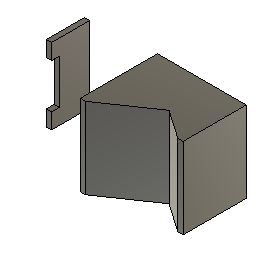
camera_enclosure v9 (Autodesk Fusion 360 design; units mm, degrees)
Autodesk Fusion 360 part; units mm, degrees
sketch "Esboço1" plane through (0, 0, 0) normal (0, 0, 1) x (1, 0, 0)
sketch "Esboço2" plane through (0, 0, 0) normal (0, 0, 1) x (1, 0, 0)
sketch "Esboço3" plane through (0, 0, 0) normal (0, 0, 1) x (1, 0, 0)
  line L0 (13, 0) -> (13, 15)
  line L1 (13, 15) -> (-13, 15)
  line L2 (-13, 15) -> (-13, 0)
  line L3 (-13, 0) -> (-13, -12)
  line L4 (-13, -12) -> (13, -12)
  line L5 (13, -12) -> (13, 0)
  constraint perpendicular L0 L1
  constraint perpendicular L3 L4
sketch "Esboço4" plane through (0, 240.56, 0) normal (0, 1, 0) x (-1, 0, 0)
  arc A0 (-80.638, 38.94) -> (-82.638, 40.94) centre (-82.638, 38.94) ccw
  line L0 (-82.638, 40.94) -> (-88.7191, 40.94)
  arc A1 (-91.2809, 40.94) -> (-88.7191, 40.94) centre (-90, 38.94) ccw
  line L1 (-91.2809, 40.94) -> (-101.2191, 40.94)
  arc A2 (-104.5, 37.6591) -> (-101.2191, 40.94) centre (-102.5, 38.94) ccw
  line L2 (-104.5, 37.6591) -> (-104.5, 19.2209)
  arc A3 (-101.2191, 15.94) -> (-104.5, 19.2209) centre (-102.5, 17.94) ccw
  line L3 (-101.2191, 15.94) -> (-91.2809, 15.94)
  arc A4 (-88.7191, 15.94) -> (-91.2809, 15.94) centre (-90, 17.94) ccw
  line L4 (-88.7191, 15.94) -> (-82.638, 15.94)
  arc A5 (-82.638, 15.94) -> (-80.638, 17.94) centre (-82.638, 17.94) ccw
  line L5 (-80.638, 17.94) -> (-80.638, 20.94)
  line L6 (-80.638, 20.94) -> (-84.238, 20.94)
  line L7 (-84.238, 20.94) -> (-84.238, 35.94)
  line L8 (-84.238, 35.94) -> (-80.638, 35.94)
  line L9 (-80.638, 35.94) -> (-80.638, 38.94)
  line L10 (-93.475, 24.965) -> (-93.475, 31.915)
  line L11 (-93.475, 31.915) -> (-86.525, 31.915)
  line L12 (-86.525, 31.915) -> (-86.525, 24.965)
  line L13 (-86.525, 24.965) -> (-93.475, 24.965)
  line L14 (-105, 42, -4) -> (-75, 42, -4)
  line L15 (-75, 42, -4) -> (-75, 15, -4)
  line L16 (-75, 15, -4) -> (-105, 15, -4)
  line L17 (-105, 15, -4) -> (-105, 42, -4)
extrude "Extrusão1" add sketch "Esboço4" against normal blind 2 contours L14 L15 L16 L17 in plane through (0, 236.56, 0) normal (0, 1, 0) makes body 1
extrude "Extrusão2" add 1 faces at (85, 234.56, 33) along direction (0, -1, 0) blind 20 on bodies 1 bodies 1
sketch "Esboço5" plane through (0, 0, 42) normal (0, 0, 1) x (-1, 0, 0)
  line L0 (-105, -236.56) -> (-75, -236.56)
  line L1 (-75, -236.56) -> (-75, -214.56)
  line L2 (-75, -214.56) -> (-105, -214.56)
  line L3 (-105, -214.56) -> (-105, -236.56)
  line L4 (-75, -222) -> (-94, -235)
  line L5 (-94, -235) -> (-105, -227.3776)
  constraint coincident L1 L4.start
  constraint coincident L3 L5.end
extrude "Extrusão3" cut sketch "Esboço5" against normal blind 29 contours L1 L2 L3 L4 L5 bodies 1
extrude "Extrusão4" add 1 faces at (81.3333, 231.1867, 42) along direction (0, 0, 1) blind 2 on bodies 1 bodies 1
extrude "Extrusão5" add 1 faces at (105, 230.4384, 34.3333) along direction (1, 0, 0) blind 2 on bodies 1 bodies 1
extrude "Extrusão6" add 1 faces at (81.3333, 231.1867, 15) along direction (0, 0, -1) blind 2 on bodies 1 bodies 1
extrude "Extrusão7" add 1 faces at (75, 231.7067, 33.6667) along direction (-1, 0, 0) blind 2 on bodies 1 bodies 1
sketch "Esboço6" plane through (0, 236.56, 0) normal (0, 1, 0) x (-1, 0, 0)
  line L0 (-73, 44) -> (-107, 44)
  line L1 (-107, 44) -> (-107, 13)
  line L2 (-107, 13) -> (-73, 13)
  line L3 (-73, 13) -> (-73, 44)
  line L4 (-105, 15) -> (-75, 15)
  line L5 (-75, 15) -> (-75, 42)
  line L6 (-75, 42) -> (-105, 42)
  line L7 (-105, 42) -> (-105, 15)
  dimension "d16" = -2
extrude "Extrusão8" add sketch "Esboço6" along normal blind 15 bodies 1
sketch "Esboço7" plane through (0, 238.96, 0) normal (0, 1, 0) x (-1, 0, 0)
  line L0 (-76.438, 20.94) -> (-76.438, 35.94)
  line L1 (-76.438, 35.94) -> (-80.638, 35.94)
  line L2 (-80.638, 35.94) -> (-80.638, 20.94)
  line L3 (-80.638, 20.94) -> (-76.438, 20.94)
  line L4 (-76.438, 35.94) -> (-76.438, 36.94)
  line L5 (-76.438, 20.94) -> (-76.438, 19.94)
  line L6 (-76.438, 19.94) -> (-71, 19.94)
  line L7 (-71, 19.94) -> (-71, 36.94)
  line L8 (-76.438, 36.94) -> (-71, 36.94)
  dimension "d19" = 1
  dimension "d20" = 1
  constraint coincident L0.end L1.start
  constraint perpendicular L1 L4
  constraint coincident L0.start L3.end
  constraint perpendicular L3 L5
  constraint perpendicular L5 L6
  constraint perpendicular L6 L7
  constraint perpendicular L7 L8
  measures "d19" distance of L0.end L4.end
  measures "d20" distance of L0.start L5.end
sketch "Esboço8" plane through (75, 0, 0) normal (1, 0, 0) x (0, 1, 0)
  line L0 (236.56, 42) -> (236.56, 15)
  line L1 (236.56, 15) -> (251.56, 15)
  line L2 (251.56, 15) -> (251.56, 42)
  line L3 (251.56, 42) -> (236.56, 42)
  line L4 (239, 20) -> (239, 37)
sketch "Esboço9" plane through (73, 0, 0) normal (-1, 0, 0) x (0, -1, 0)
  line L0 (-222, 13) -> (-222, 44)
  line L1 (-222, 44) -> (-251.56, 44)
  line L2 (-251.56, 44) -> (-251.56, 13)
  line L3 (-251.56, 13) -> (-222, 13)
  line L4 (-239, 37) -> (-236, 37)
  line L5 (-236, 37) -> (-236, 20)
  line L6 (-236, 20) -> (-239, 20)
  line L7 (-239, 20) -> (-239, 37)
  dimension "d23" = 3
  constraint perpendicular L0 L4
  constraint perpendicular L4 L5
  constraint perpendicular L5 L6
  constraint perpendicular L4 L7
  measures "d23" distance of L4.start L4.end
extrude "Extrusão9" cut sketch "Esboço9" against normal blind 2 contours L4 L5 L6 L7 bodies 1
sketch "Esboço10" plane through (0, 0, 42) normal (0, 0, -1) x (1, 0, 0)
  line L0 (105, -236.56) -> (75, -236.56)
  line L1 (75, -236.56) -> (75, -251.56)
  line L2 (75, -251.56) -> (105, -251.56)
  line L3 (105, -251.56) -> (105, -236.56)
  line L4 (105, -250.56) -> (105, -249.56)
  line L5 (105, -250.56) -> (75, -250.56)
  line L6 (75, -250.56) -> (75, -249.56)
  line L7 (75, -249.56) -> (105, -249.56)
  dimension "d27" = 1
  dimension "d28" = 1
  dimension "d29" = 90
  dimension "d30" = 1
  constraint parallel L3 L4
  constraint coincident L1 L5.end
  constraint perpendicular L5 L6
  measures "d27" distance of L2.end L4.start
  measures "d28" distance of L4.start L4.end
  measures "d29" angle of L4 L5
  measures "d30" distance of L5.end L6.end
extrude "Extrusão10" add sketch "Esboço10" along normal blind 28 contours L1 L3 L4 L5 L6 L7 bodies 1
sketch "Esboço11" plane through (0, 250.56, 0) normal (0, 1, 0) x (-1, 0, 0)
  line L0 (-105, 15) -> (-75, 15)
  line L1 (-75, 15) -> (-75, 42)
  line L2 (-75, 42) -> (-105, 42)
  line L3 (-105, 42) -> (-105, 15)
  line L4 (-103, 17) -> (-77, 17)
  line L5 (-77, 17) -> (-77, 40)
  line L6 (-77, 40) -> (-103, 40)
  line L7 (-103, 40) -> (-103, 17)
  dimension "d33" = -2
extrude "Extrusão11" cut sketch "Esboço11" against normal blind 1 contours L4 L5 L6 L7 bodies 1
sketch "Esboço12" plane through (0, 251.56, 0) normal (0, 1, 0) x (-1, 0, 0)
  line L0 (-105, 15) -> (-105, 42)
  line L1 (-105, 42) -> (-75, 42)
  line L2 (-75, 42) -> (-75, 15)
  line L3 (-75, 15) -> (-105, 15)
  line L4 (-73, 13) -> (-73, 44)
  line L5 (-73, 44) -> (-107, 44)
  line L6 (-107, 44) -> (-107, 13)
  line L7 (-107, 13) -> (-73, 13)
  line L8 (-105, 42) -> (-75, 42)
  line L9 (-75, 42) -> (-75, 15)
  line L10 (-75, 15) -> (-105, 15)
  line L11 (-105, 15) -> (-105, 42)
  circle A0 centre (-90, 28.5) radius 3.6401
  constraint horizontal L8
  constraint vertical L9
  constraint horizontal L10
  constraint vertical L11
  constraint coincident L2.end L3.start
  constraint coincident L0.end L1.start
extrude "Extrusão1'" add sketch "Esboço12" along normal blind 1 separate body contours L0 L1 L2 L3 L8 L9 L10 L11 makes body 2 in component "Component"
combine "Combinar1" operation add target body 2 tool bodies 1 body 1 seen with x (1, 0, 0) y (0, 1, 0) z (0, 0, 1) at (0, 1, 0) in component "Component"
sketch "Esboço13" plane through (0, 0, 44) normal (0, 0, 1) x (-1, 0, 0)
  line L0 (-94, -235) -> (-105, -227.3776)
  line L1 (-105, -227.3776) -> (-107, -227.3776)
  line L2 (-107, -227.3776) -> (-107, -251.56)
  line L3 (-107, -251.56) -> (-73, -251.56)
  line L4 (-73, -251.56) -> (-73, -222)
  line L5 (-73, -222) -> (-75, -222)
  line L6 (-75, -222) -> (-94, -235)
sketch "Esboço14" plane through (73, 0, 0) normal (-1, 0, 0) x (0, -1, 0)
  line L0 (-236, 37) -> (-236, 20)
  line L1 (-236, 20) -> (-239, 20)
  line L2 (-239, 20) -> (-239, 37)
  line L3 (-239, 37) -> (-236, 37)
  line L4 (-222, 13) -> (-222, 44)
  line L5 (-222, 44) -> (-251.56, 44)
  line L6 (-251.56, 44) -> (-251.56, 13)
  line L7 (-251.56, 13) -> (-222, 13)
  line L8 (-250.56, 14) -> (-223, 14)
  line L9 (-223, 14) -> (-223, 43)
  line L10 (-223, 43) -> (-250.56, 43)
  line L11 (-250.56, 43) -> (-250.56, 14)
  line L12 (-236, 37) -> (-236, 43)
  line L13 (-236, 20) -> (-236, 14)
  dimension "d38" = -1
  constraint coincident L0.start L3.end
  constraint coincident L10 L12.end
  constraint perpendicular L10 L12
  constraint coincident L0.end L1.start
  constraint coincident L8 L13.end
  constraint perpendicular L8 L13
extrude "Extrusão2'" cut sketch "Esboço14" against normal blind 1 contours L1 L2 L3 L8 L10 L11 L12 L13 sketch seen with x (1, 0, 0) y (0, 1, 0) z (0, 0, 1) at (0, 1, 0) bodies 2 in component "Component"
extrude "Extrusão3'" cut 1 faces at (74, 247.7067, 25.6667) along direction (1, 0, 0) blind 1 on bodies 2 bodies 2 in component "Component"
sketch "Esboço15" plane through (75, 0, 0) normal (-1, 0, 0) x (0, -1, 0)
  line L0 (-236.56, 42) -> (-236.56, 15)
  line L1 (-236.56, 15) -> (-249.56, 15)
  line L2 (-249.56, 15) -> (-249.56, 42)
  line L3 (-249.56, 42) -> (-236.56, 42)
  line L4 (-236, 14) -> (-236, 43)
  line L5 (-236, 43) -> (-250.56, 43)
  line L6 (-250.56, 43) -> (-250.56, 14)
  line L7 (-250.56, 14) -> (-236, 14)
  line L8 (-239, 37) -> (-236, 37)
  line L9 (-239, 21) -> (-236, 21)
  line L10 (-236, 21) -> (-236, 37)
  constraint coincident L4 L8.end
  constraint perpendicular L4 L8
  constraint coincident L4 L9.end
  constraint perpendicular L4 L9
extrude "Extrusão1''" add sketch "Esboço15" along normal blind 2 separate body contours L0 L1 L2 L3 L4 L5 L6 L7 L8 L9 | L0 L1 L2 L3 makes body 3 in component "Component'"
sketch "Esboço16" plane through (73, 0, 0) normal (-1, 0, 0) x (0, -1, 0)
  line L0 (-236, 37) -> (-236, 43)
  line L1 (-236, 43) -> (-250.56, 43)
  line L2 (-250.56, 43) -> (-250.56, 14)
  line L3 (-250.56, 14) -> (-236, 14)
  line L4 (-236, 14) -> (-236, 21)
  line L5 (-236, 21) -> (-236.56, 21)
  line L6 (-236.56, 21) -> (-236.56, 37)
  line L7 (-236.56, 37) -> (-236, 37)
  line L8 (-236.56, 37) -> (-239, 37)
  line L9 (-239, 20) -> (-236, 20)
  line L10 (-236, 20) -> (-236, 37)
  line L11 (-236, 37) -> (-236.56, 37)
  line L12 (-239, 37) -> (-239, 20)
  constraint coincident L6.end L7.start
  constraint perpendicular L6 L8
  constraint coincident L4 L9.end
  constraint perpendicular L4 L9
  constraint coincident L0.start L7.end
  constraint perpendicular L9 L12
extrude "Extrusão2''" cut sketch "Esboço16" against normal blind 2 contours L4 L5 L6 L8 L9 L10 L12 bodies 3 in component "Component'"
component "Component" placed x (1, 0, 0) y (0, 1, 0) z (0, 0, 1) at (0, -1, 0)
component "Component'" placed x (1, 0, 0) y (0, 1, 0) z (0, 0, 1) at (0, 0, 0)
